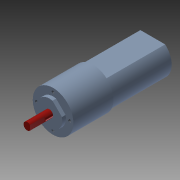
# Autodesk Inventor part: Motor
Saved by Autodesk Inventor 2016 (Build 200138000, 138)
## iProperties
Created: 2013-02-22
Part Number: Motor
Material: Generic
Document SubType Name: Modeling
Designer: lk8187
Density: 1 g/cm^3
Appearance: Light Steel Blue
Author: lk8187
Autodesk Inventor part; units mm, degrees
ref_plane "YZ Plane" through (0, 0, 0) normal (1, 0, 0) x (0, 1, 0)
ref_plane "XZ Plane" through (0, 0, 0) normal (0, 1, 0) x (-1, 0, 0)
ref_plane "XY Plane" through (0, 0, 0) normal (0, 0, 1) x (1, 0, 0)
sketch "Sketch1" plane through (0, 0, 0) normal (1, 0, 0) x (0, 1, 0)
  line L0 (0, 0) -> (-9.28, 0)
  line L1 (0, 0) -> (0, 2)
  line L2 (0, 2) -> (12, 2)
  line L3 (12, 2) -> (12, 7)
  line L4 (12, 7) -> (14, 7)
  line L5 (14, 7) -> (14, 11)
  line L6 (14, 11) -> (35.7, 11)
  line L7 (35.7, 11) -> (35.7, 10.25)
  line L8 (35.7, 10.25) -> (68, 10.25)
  line L9 (68, 10.25) -> (68, 0)
  line L10 (68, 0) -> (0, 0)
  dimension "d0" = 4
  dimension "d2" = 12
  dimension "d3" = 2
  dimension "d5" = 22
  dimension "d6" = 20.5
  dimension "d7" = 32.3
  dimension "d8" = 21.7
  dimension "d32" = 14
  constraints: 22 end point, 7 parallel, 2 perpendicular, 1 collinear, 1 horizontal
  measures "d0" diameter of L2 L0
  measures "d2" distance between parallel lines of L1 L3
  measures "d3" distance of L3.end L4.end
  measures "d5" diameter of L6 L0
  measures "d6" diameter of L8 L0
  measures "d7" distance between parallel lines of L9 L7
  measures "d8" distance between parallel lines of L5 L7
  measures "d32" diameter of L4 L0
revolve "Revolution1" add sketch "Sketch1" angle 360 about axis through (0, 0, 0) along (0, -1, 0)
sketch "Sketch2" plane through (0, 14, 0) normal (0, -1, 0) x (1, 0, 0)
  circle A0 centre (0, 0) radius 11 projected
  point P0 (0, 9)
  point P1 (-9, 0)
  point P2 (0, -9)
  point P3 (9, 0)
  dimension "d12" = 360
  dimension "d15" = 18
  constraints: 1 vertical alignment, 5 other
  measures "d15" distance of point (-9, 0) point (9, 0)
hole "Hole1" at (0, 14, 9) at (-9, 14, 0) at (0, 14, -9) at (9, 14, 0) direction (0, 1, 0) diameter 1.567 depth 4 tip angle 118 thread size "M2x0.4" class "6H" standard "ANSI Metric M Profile"
sketch "Sketch3" plane through (0, 12, 0) normal (0, -1, 0) x (1, 0, 0)
  circle A0 centre (0, 0) radius 7 projected
  circle A1 centre (0, 0) radius 2 projected
  line L0 (1.6931, 6.7922) -> (6.7922, 1.6931)
  line L1 (-1.6931, -6.7922) -> (-6.7922, -1.6931)
  line L2 (0, 0) -> (-24.8191, 0) construction
  dimension "d23" = 135
  dimension "d24" = 12
  constraints: 6 end point, 4 point on circle, 2 parallel, 1 horizontal
  measures "d23" angle of L2 L1
  measures "d24" distance between parallel lines of L1 L0
extrude "Extrusion1" cut sketch "Sketch3" against normal up to surface (2 mm away) contours L0 A0 | A0 L1
sketch "Sketch4" plane through (0, 0, 0) normal (0, -1, 0) x (1, 0, 0)
  circle A0 centre (0, 0) radius 2 projected
  line L0 (1.5, 1.3229) -> (1.5, -1.3229)
  dimension "d28" = 1.5
  constraints: 2 end point, 2 point on circle, 1 vertical
  measures "d28" distance from line of A0.centre L0
extrude "Extrusion2" cut sketch "Sketch4" against normal blind 8 contours A0 L0 picked at (1.5908, -0.3089)
sketch "Sketch5" plane through (0, 68, 0) normal (0, 1, 0) x (1, 0, 0)
  circle A0 centre (0, 0) radius 10.25 projected
  line L0 (-6.7082, 7.75) -> (6.7082, 7.75)
  line L1 (6.7082, -7.75) -> (-6.7082, -7.75)
  dimension "d33" = 15.5
  constraints: 4 end point, 4 point on circle, 2 parallel, 1 horizontal
  measures "d33" distance between parallel lines of L0 L1
extrude "Extrusion3" cut sketch "Sketch5" against normal up to surface (32.3 mm away) contours L0 A0 | A0 L1
body "Solid1"
